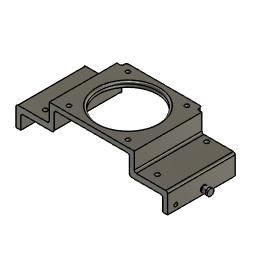
FS80+UL Bracket v17 (Autodesk Fusion 360 design; units mm, degrees)
Autodesk Fusion 360 part; units mm, degrees
sketch "Schizzo1" plane through (0, 0, 0) normal (0, 0, 1) x (1, 0, 0)
  line L0 (-32.4508, 65.6855) -> (45.5492, 65.6855)
  line L1 (45.5492, 65.6855) -> (45.5492, -9.3145)
  line L2 (45.5492, -9.3145) -> (-32.4508, -9.3145)
  line L3 (-32.4508, -9.3145) -> (-32.4508, 65.6855)
  line L4 (-32.4508, 28.1855) -> (45.5492, 28.1855) construction
  line L5 (6.5492, 65.6855) -> (6.5492, -9.3145) construction
  circle A0 centre (6.5492, 28.1855) radius 30.5
  line L6 (37.0492, -2.3145) -> (-23.9508, -2.3145) construction
  line L7 (-23.9508, -2.3145) -> (-23.9508, 58.6855) construction
  line L8 (-23.9508, 58.6855) -> (37.0492, 58.6855) construction
  line L9 (37.0492, 58.6855) -> (37.0492, -2.3145) construction
  line L10 (37.0492, -2.3145) -> (-23.9508, 58.6855) construction
  line L11 (-23.9508, -2.3145) -> (37.0492, 58.6855) construction
  circle A1 centre (-23.9508, 58.6855) radius 2.1
  circle A2 centre (37.0492, 58.6855) radius 2.1
  circle A3 centre (37.0492, -2.3145) radius 2.1
  circle A4 centre (-23.9508, -2.3145) radius 2.1
  line L12 (-71.9508, 58.6855) -> (-66.9508, 58.6855)
  line L13 (-66.9508, 58.6855) -> (-66.9508, -2.3145)
  line L14 (-66.9508, -2.3145) -> (-71.9508, -2.3145)
  line L15 (-71.9508, -2.3145) -> (-71.9508, 58.6855)
  line L16 (85.0492, 58.6855) -> (80.0492, 58.6855)
  line L17 (85.0492, -2.3145) -> (85.0492, 58.6855)
  line L18 (80.0492, 58.6855) -> (80.0492, -2.3145)
  line L19 (80.0492, -2.3145) -> (85.0492, -2.3145)
  circle A5 centre (-23.9508, 58.6855) radius 3.6
  circle A6 centre (37.0492, 58.6855) radius 3.6
  circle A7 centre (-23.9508, -2.3145) radius 3.6
  circle A8 centre (37.0492, -2.3145) radius 3.6
  line L20 (-32.4508, -9.3145) -> (-71.9508, -9.3145)
  line L21 (-71.9508, -9.3145) -> (-71.9508, -2.3145)
  line L22 (45.5492, -9.3145) -> (85.0492, -9.3145)
  line L23 (85.0492, -9.3145) -> (85.0492, -2.3145)
  line L24 (-66.9508, -2.3145) -> (-66.9508, -9.3145)
  line L25 (80.0492, -2.3145) -> (80.0492, -9.3145)
  line L26 (-66.9508, 58.6855) -> (-32.4508, 58.6855)
  line L27 (80.0492, 58.6855) -> (45.5492, 58.6855)
  line L28 (-66.9508, 58.6855) -> (-32.4508, 58.6855)
  line L29 (-32.4508, 58.6855) -> (-32.4508, 60.6855)
  line L30 (-32.4508, 60.6855) -> (-66.9508, 60.6855)
  line L31 (-66.9508, 60.6855) -> (-66.9508, 58.6855)
  line L32 (80.0492, 60.6855) -> (80.0492, 58.6855)
  line L33 (45.5492, 60.6855) -> (80.0492, 60.6855)
  line L34 (80.0492, 58.6855) -> (45.5492, 58.6855)
  line L35 (45.5492, -9.3145) -> (45.5492, 65.6855)
  line L36 (-37.4508, -9.3145) -> (-37.4508, 60.6855)
  line L37 (50.5492, -9.3145) -> (50.5492, 60.6855)
  line L38 (-71.9508, 58.6855) -> (-66.9508, 58.6855)
  line L39 (-66.9508, 58.6855) -> (-66.9508, 60.6855)
  line L40 (-66.9508, 60.6855) -> (-71.9508, 60.6855)
  line L41 (-71.9508, 60.6855) -> (-71.9508, 58.6855)
  line L42 (85.0492, 60.6855) -> (85.0492, 58.6855)
  line L43 (80.0492, 60.6855) -> (85.0492, 60.6855)
  point P0 (6.5492, 28.1855)
  point P1 (-23.9508, -2.3145)
  dimension "d1" = 78
  dimension "d2" = 75
  dimension "d3" = 61
  dimension "d4" = 61
  dimension "d5" = 61
  dimension "d6" = 4.2
  dimension "d13" = 5
  dimension "d22" = 7.2
  dimension "d70" = 157
  dimension "d82" = 147
  dimension "d102" = 2
  dimension "d109" = 5
  constraint horizontal L0
  constraint vertical L1
  constraint horizontal L2
  constraint vertical L3
  constraint midpoint L3 L4.start
  constraint midpoint L1 L4.end
  constraint midpoint L0 L5.start
  constraint midpoint L2 L5.end
  constraint midpoint L4 P0
  constraint horizontal L6
  constraint perpendicular L6 L7
  constraint parallel L6 L8
  constraint parallel L7 L9
  constraint coincident L10 P0
  constraint coincident L11 P0
  constraint coincident P0 A0.centre
  constraint coincident L7.end L8.start
  constraint symmetric L5 A1 A2
  constraint symmetric L4 L7.end P1
  constraint symmetric L4 A2 A3
  constraint symmetric L4 A1 A4
  constraint horizontal L12
  constraint vertical L13
  constraint horizontal L14
  constraint vertical L15
  constraint collinear L8 L12
  constraint collinear L6 L14
  constraint symmetric L5 L12.start L16.start
  constraint symmetric L5 L12.end L16.end
  constraint symmetric L5 L13.end L18.end
  constraint symmetric L5 L14.end L17.start
  constraint concentric A1 A5
  constraint symmetric L5 A5 A6
  constraint symmetric L4 A5 A7
  constraint symmetric L4 A6 A8
  constraint horizontal L20
  constraint vertical L21
  constraint horizontal L22
  constraint vertical L23
  constraint coincident L20 L24.end
  constraint perpendicular L20 L24
  constraint symmetric L5 L24.end L25.end
  constraint coincident L3 L26.end
  constraint perpendicular L3 L26
  constraint symmetric L5 L26.end L27.end
  constraint horizontal L28
  constraint vertical L29
  constraint horizontal L30
  constraint vertical L31
  constraint collinear L3 L29
  constraint symmetric L0.start L5 L0.end
  constraint symmetric L2.end L5 L1.end
  constraint symmetric L5 L29.end L33.start
  constraint symmetric L5 L30.end L32.start
  constraint coincident L20 L36.start
  constraint coincident L30 L36.end
  constraint perpendicular L30 L36
  constraint symmetric L5 L36.start L37.start
  constraint symmetric L5 L36.end L37.end
  constraint horizontal L38
  constraint vertical L39
  constraint horizontal L40
  constraint vertical L41
  constraint symmetric L5 L40.end L42.start
  measures "d1" distance of L0.start L0.end
  measures "d2" distance of L0.start L2.end
  measures "d3" diameter of A0
  measures "d4" distance of L7.end L8.end
  measures "d5" distance of P1 L7.end
  measures "d6" diameter of A1
  measures "d13" distance of L13 L15
  measures "d22" diameter of A5
  measures "d70" distance of L15 L17
  measures "d82" distance of L13 L18
  measures "d102" distance of L28 L30
  measures "d109" distance of L3 L36
extrude "Estrusione1" add sketch "Schizzo1" along normal blind 5 contours L0 L1 L2 L3 L29 L35 | L3 L26 L28 L29 L30 L36 | L1 L27 L33 L34 L35 L37 | L3 L20 L26 L28 L36 | L1 L22 L27 L34 L35 L37 | A5 | A6 | A7 | A8
fillet "Raccordo22" radius 2 1 edges at (-21.8868, 39.2148, 5)
extrude "Estrusione14" add sketch "Schizzo1" against normal blind 20 contours L3 L26 L28 L29 L30 L36 | L1 L27 L33 L34 L35 L37 | L3 L20 L26 L28 L36 | L1 L22 L27 L34 L35 L37
fillet "Raccordo20" radius 2 2 edges at (-32.4508, 25.6855, 0) (45.5492, 25.6855, 0)
fillet "Raccordo17" radius 2 2 edges at (-32.4508, 65.6855, 2.5) (45.5492, 65.6855, 2.5)
fillet "Raccordo21" radius 2 2 edges at (45.5492, 60.6855, 2.5) (-32.4508, 60.6855, 2.5)
extrude "Estrusione15" add sketch "Schizzo1" along normal blind 6 from surface at -20 contours L3 L20 L26 L28 L36 | L26 L28 L30 L31 L36 L39 | L1 L22 L27 L34 L35 L37 | L27 L32 L33 L34 L37 | L13 L20 L24 L26 L28 L36 | L12 L31 L38 L39 L40 L41 | L18 L22 L25 L27 L34 L37 | L16 L32 L42 L43 | L12 L13 L14 L15 L38 | L16 L17 L18 L19 | L14 L20 L21 L24 | L19 L22 L23 L25
fillet "Raccordo14" radius 2 2 edges at (50.5492, 25.6855, -14) (-37.4508, 25.6855, -14)
fillet "Raccordo18" radius 2 2 edges at (45.5492, 25.6855, -20) (-32.4508, 25.6855, -20)
extrude "Estrusione2" add sketch "Schizzo1" against normal blind 20 from surface at -15 contours L12 L31 L38 L39 L40 L41 | L16 L32 L42 L43 | L12 L13 L14 L15 L38 | L16 L17 L18 L19 | L14 L20 L21 L24 | L19 L22 L23 L25
fillet "Raccordo23" radius 2 2 edges at (-71.9508, 25.6855, -14) (85.0492, 25.6855, -14)
fillet "Raccordo24" radius 2 2 edges at (-66.9508, 25.6855, -20) (80.0492, 25.6855, -20)
sketch "Schizzo2" plane through (-71.9508, 0, 0) normal (-1, 0, 0) x (0, -1, 0)
  line L0 (-60.6855, -35) -> (9.3145, -35)
  circle A0 centre (-28.1855, -30) radius 2.9
  circle A1 centre (-28.1855, -30) radius 3.5
  line L1 (9.3145, -35) -> (9.3145, -16)
  circle A2 centre (0.8145, -30) radius 1.9
  line L2 (-58.6855, -15) -> (9.3145, -15) construction
  line L3 (9.3145, -15) -> (9.3145, -35) construction
  line L4 (9.3145, -35) -> (-58.6855, -35) construction
  line L5 (-58.6855, -35) -> (-58.6855, -15) construction
  line L6 (-58.6855, -30) -> (9.3145, -30) construction
  line L7 (9.3145, -16) -> (-60.6855, -16)
  line L8 (-60.6855, -16) -> (-60.6855, -35)
  dimension "d27" = 5.8
  dimension "d28" = 7
  dimension "d56" = 3.8
  dimension "d94" = 5
  dimension "d95" = 30.5
  dimension "d96" = 29
  constraint coincident A0.centre A1.centre
  constraint horizontal L2
  constraint vertical L3
  constraint horizontal L4
  constraint vertical L5
  constraint collinear L0 L4
  constraint collinear L1 L3
  constraint coincident L5 L6.start
  constraint coincident L3 L6.end
  constraint perpendicular L3 L6
  constraint coincident A0.centre L6
  constraint coincident A2.centre L6
  measures "d27" diameter of A0
  measures "d28" diameter of A1
  measures "d56" diameter of A2
  measures "d94" distance of L4 L6
  measures "d95" distance of A0.centre L5
  measures "d96" distance of A0.centre A2.centre
extrude "Estrusione4" add sketch "Schizzo2" along normal blind 7 contours A0
extrude "Estrusione5" add sketch "Schizzo2" against normal blind 2 from surface at 7 contours A1
fillet "Raccordo4" radius 0.5 1 edges at (-71.9508, 30.8893, -28.9513)
extrude "Estrusione10" cut sketch "Schizzo2" against normal blind 3.5 contours A2
sketch "Schizzo3" plane through (85.0492, 0, 0) normal (1, 0, 0) x (0, 1, 0)
  line L0 (-9.3145, -35) -> (60.6855, -35)
  circle A0 centre (28.1855, -30) radius 2.9
  circle A1 centre (28.1855, -30) radius 3.5
  circle A2 centre (-0.8145, -30) radius 1.9
  line L1 (-9.3145, -16) -> (-9.3145, -35)
  line L2 (58.6855, -35) -> (-9.3145, -35) construction
  line L3 (-9.3145, -35) -> (-9.3145, -15) construction
  line L4 (-9.3145, -15) -> (58.6855, -15) construction
  line L5 (58.6855, -15) -> (58.6855, -35) construction
  line L6 (-9.3145, -30) -> (58.6855, -30) construction
  line L7 (60.6855, -16) -> (-9.3145, -16)
  line L8 (60.6855, -35) -> (60.6855, -16)
  dimension "d36" = 5.8
  dimension "d37" = 7
  dimension "d49" = 3.8
  dimension "d97" = 5
  dimension "d98" = 29
  dimension "d99" = 30.5
  constraint concentric A0 A1
  constraint horizontal L2
  constraint vertical L3
  constraint horizontal L4
  constraint vertical L5
  constraint collinear L0 L2
  constraint collinear L1 L3
  constraint coincident L1 L6.start
  constraint coincident L5 L6.end
  constraint perpendicular L5 L6
  constraint coincident A2.centre L6
  constraint coincident A0.centre L6
  measures "d36" diameter of A0
  measures "d37" diameter of A1
  measures "d49" diameter of A2
  measures "d97" distance of L2 L6
  measures "d98" distance of A0.centre A2.centre
  measures "d99" distance of A0.centre L5
extrude "Estrusione6" add sketch "Schizzo3" along normal blind 7 contours A0
extrude "Estrusione7" add sketch "Schizzo3" against normal blind 2 from surface at 7 contours A1
fillet "Raccordo5" radius 0.5 1 edges at (85.0492, 25.4818, -28.9513)
extrude "Estrusione11" cut sketch "Schizzo3" against normal blind 3.5 contours A2
sketch "Schizzo4" plane through (0, 0, 5) normal (0, 0, 1) x (-1, 0, 0)
  line L0 (37.4508, 9.3145) -> (-50.5492, 9.3145)
  line L1 (-43.5492, -65.6855) -> (30.4508, -65.6855)
  circle A0 centre (23.9508, 2.3145) radius 2.1
  circle A1 centre (-37.0492, -58.6855) radius 2.1
  circle A2 centre (23.9508, -58.6855) radius 2.1
  circle A3 centre (-37.0492, 2.3145) radius 2.1
  line L2 (65.9508, -65.6855) -> (-79.0492, -65.6855) construction
  line L3 (-79.0492, -65.6855) -> (-79.0492, 9.3145) construction
  line L4 (-79.0492, 9.3145) -> (65.9508, 9.3145) construction
  line L5 (65.9508, 9.3145) -> (65.9508, -65.6855) construction
  line L6 (-6.5492, -65.6855) -> (-6.5492, 9.3145) construction
  line L7 (-6.5492, -28.1855) -> (65.9508, -28.1855) construction
  line L8 (-6.5492, -28.1855) -> (-79.0492, -28.1855) construction
  line L9 (65.9508, -55.6855) -> (-79.0492, -55.6855) construction
  line L10 (65.9508, -0.6855) -> (-79.0492, -0.6855) construction
  circle A4 centre (47.4508, -55.6855) radius 2.25
  circle A5 centre (47.4508, -55.6855) radius 3.75
  circle A6 centre (51.4508, -0.6855) radius 2.25
  circle A7 centre (51.4508, -0.6855) radius 3.75
  circle A8 centre (-60.5492, -55.6855) radius 2.25
  circle A9 centre (-60.5492, -55.6855) radius 3.75
  circle A10 centre (-64.5492, -0.6855) radius 3.75
  circle A11 centre (-64.5492, -0.6855) radius 2.25
  line L11 (-45.5492, -62.6855) -> (-45.5492, -63.6855)
  line L12 (32.4508, -63.6855) -> (32.4508, -62.6855)
  line L13 (-50.5492, 9.3145) -> (-50.5492, -60.6855)
  line L14 (37.4508, -60.6855) -> (37.4508, 9.3145)
  arc A12 (-45.5492, -63.6855) -> (-43.5492, -65.6855) centre (-43.5492, -63.6855) ccw
  arc A13 (30.4508, -65.6855) -> (32.4508, -63.6855) centre (30.4508, -63.6855) ccw
  circle A14 centre (-6.5492, -28.1855) radius 32.5
  arc A15 (34.4508, -60.6855) -> (32.4508, -62.6855) centre (34.4508, -62.6855) ccw
  line L15 (34.4508, -60.6855) -> (37.4508, -60.6855)
  line L16 (-50.5492, -60.6855) -> (-47.5492, -60.6855)
  arc A16 (-45.5492, -62.6855) -> (-47.5492, -60.6855) centre (-47.5492, -62.6855) ccw
  point P0 (47.4508, -55.6855)
  point P1 (51.4508, -0.6855)
  point P2 (-60.5492, -55.6855)
  point P3 (-64.5492, -0.6855)
  dimension "d79" = 55
  dimension "d80" = 108
  dimension "d81" = 116
  dimension "d83" = 4.5
  dimension "d84" = 7.5
  dimension "d85" = 4.5
  dimension "d86" = 7.5
  constraint horizontal L2
  constraint vertical L3
  constraint horizontal L4
  constraint vertical L5
  constraint collinear L1 L2
  constraint collinear L0 L4
  constraint midpoint L2 L6.start
  constraint midpoint L4 L6.end
  constraint midpoint L5 L7.end
  constraint midpoint L3 L8.end
  constraint perpendicular L6 L9
  constraint symmetric L8 L9.start L10.start
  constraint symmetric L8 L9.end L10.end
  constraint coincident L5 L9.start
  constraint coincident L3 L9.end
  constraint coincident L9 P0
  constraint coincident L10 P1
  constraint symmetric L6 P0 P2
  constraint symmetric L6 P1 P3
  constraint coincident P0 A4.centre
  constraint concentric A4 A5
  constraint coincident P1 A6.centre
  constraint symmetric L6 A4 A8
  constraint symmetric L6 A5 A9
  constraint symmetric L6 A6 A11
  constraint symmetric L6 A7 A10
  measures "d79" distance of L9 L10
  measures "d80" distance of P0 P2
  measures "d81" distance of P1 P3
  measures "d83" diameter of A4
  measures "d84" diameter of A5
  measures "d85" diameter of A6
  measures "d86" diameter of A7
extrude "Estrusione12" cut sketch "Schizzo4" against normal blind 6 from surface at -19 contours A4 | A6 | A8 | A11
equation "d1 = 75 mm + 0.2 mm + 2.8 mm"
equation "d85 = d83"
equation "d86 = d84"
